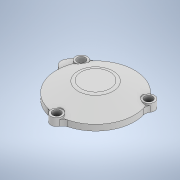
# Autodesk Inventor part: 64. Крышка подшипника
Saved by Autodesk Inventor 2021 (Build 250183000, 183)
## iProperties
Created: 2021-03-10
Part Number: 64. Крышка подшипника
Material: Типовые
Document SubType Name: Modeling
Designer: Данил
Density: 1 g/cm^3
Appearance: По умолчанию
Author: Данил
Autodesk Inventor part; units mm, degrees
ref_plane "YZ Plane" through (0, 0, 0) normal (1, 0, 0) x (0, 1, 0)
ref_plane "XZ Plane" through (0, 0, 0) normal (0, 1, 0) x (-1, 0, 0)
ref_plane "XY Plane" through (0, 0, 0) normal (0, 0, 1) x (1, 0, 0)
sketch "Эскиз1" plane through (0, 0, 0) normal (0, 0, 1) x (1, 0, 0)
  line L0 (0, 11.25) -> (0, -11.25)
  line L1 (-44, -11.25) -> (-44, -8.6)
  line L2 (-42, -6.6) -> (-33.5, -6.6)
  line L3 (-33.5, -6.6) -> (-33.5, -3.25)
  line L4 (-44, -11.25) -> (-53, -11.25)
  line L5 (-53, -11.25) -> (-53, -3.25)
  line L6 (-53, -3.25) -> (-23.9139, 10.3131)
  arc A0 (-42, -6.6) -> (-44, -8.6) centre (-42, -8.6) ccw
  line L7 (-19.6877, 6.75) -> (0, 6.75)
  line L8 (-19.6877, 11.25) -> (0, 11.25)
  arc A1 (-19.6877, 11.25) -> (-23.9139, 10.3131) centre (-19.6877, 1.25) ccw
  line L9 (-30.5721, 1.9039) -> (-24.8078, 5.3398)
  arc A2 (-30.5721, 1.9039) -> (-33.5, -3.25) centre (-27.5, -3.25) ccw
  arc A3 (-19.6877, 6.75) -> (-24.8078, 5.3398) centre (-19.6877, -3.25) ccw
  point P0 (0, 0)
  point P1 (0, 0)
  dimension "d0" = 22.5
  dimension "d1" = 88
  dimension "d2" = 67
  dimension "d3" = 4.65
  dimension "d4" = 2
  dimension "d6" = 8
  dimension "d7" = 106
  dimension "d8" = 25
  dimension "d9" = 4.5
  dimension "d10" = 10
  dimension "d11" = 6
  dimension "d12" = 10
  constraints: 20 end point, 8 point on circle, 8 tangent, 4 centre point, 3 coincident, 3 horizontal, 3 perpendicular, 2 horizontal alignment, 2 vertical, 2 vertical alignment, 1 midpoint
  measures "d0" distance of L0.start L0.end
  measures "d1" diameter of L1 L0
  measures "d2" diameter of L3 L0
  measures "d3" distance between parallel lines of L2 L4
  measures "d4" radius of A0
  measures "d6" distance from line of L4 L5.end
  measures "d7" diameter of L5 L0
  measures "d8" angle of L6 L8
  measures "d9" distance between parallel lines of L7 L8
  measures "d10" radius of A1
  measures "d11" radius of A2
  measures "d12" radius of A3
revolve "Вращение1" add sketch "Эскиз1" angle 360 about axis through (0, 11.25, 0) along (0, -1, 0)
sketch "Эскиз2" plane through (0, -11.25, 0) normal (0, -1, 0) x (1, 0, 0)
  circle A0 centre (0, 0) radius 53 projected
  arc A1 (-13.6119, 51.2222) -> (-7.1912, 56.5052) centre (-16.1802, 60.8868) ccw
  arc A2 (7.1912, 56.5052) -> (13.6119, 51.2222) centre (16.1802, 60.8868) ccw
  circle A3 centre (0, 53) radius 8
  arc A4 (51.1657, -13.8229) -> (52.5306, -22.0249) centre (60.8196, -16.4309) ccw
  arc A5 (45.3394, -34.4804) -> (37.5538, -37.3994) centre (44.6394, -44.4559) ccw
  circle A6 centre (45.8993, -26.5) radius 8
  line L0 (0, 0) -> (45.8993, -26.5) construction
  line L1 (0, 0) -> (0, 53) construction
  line L2 (0, 0) -> (-45.8993, -26.5) construction
  arc A7 (-37.5538, -37.3994) -> (-45.3394, -34.4804) centre (-44.6394, -44.4559) ccw
  circle A8 centre (-45.8993, -26.5) radius 8
  line L3 (-52.7372, -30.6525) -> (-59.6376, -19.2897)
  arc A9 (-55.6932, -5.2214) -> (-52.9952, -0.7151) centre (-57.9947, -0.7826) ccw
  arc A10 (-55.6932, -5.2214) -> (-59.6376, -19.2897) centre (-51.0903, -14.099) ccw
  point P0 (0, 0)
  point P1 (-49.3651, -19.2897)
  dimension "d14" = 10
  dimension "d15" = 10
  dimension "d16" = 16
  dimension "d17" = 16
  dimension "d18" = 10
  dimension "d19" = 10
  dimension "d20" = 120
  dimension "d21" = 120
  dimension "d22" = 16
  dimension "d24" = 10
  dimension "d25" = 5
  dimension "d26" = 10
  constraints: 21 point on circle, 10 centre point, 8 end point, 8 tangent, 2 coincident, 1 horizontal alignment, 1 vertical, 1 vertical alignment, 18 other
  measures "d14" radius of A2
  measures "d15" radius of A1
  measures "d16" diameter of A3
  measures "d17" diameter of A6
  measures "d18" radius of A4
  measures "d19" radius of A5
  measures "d20" angle of L1 L0
  measures "d21" angle of L2 L1
  measures "d22" diameter of A8
  measures "d24" radius of A7
  measures "d25" radius of A9
  measures "d26" radius of A10
extrude "Выдавливание1" add sketch "Эскиз2" against normal blind 8 contours A0 A3 A2 | A4 A6 A0 | A0 A3 | A6 A0 | A0 A1 A3 | A6 A5 A0 | A0 A8 L3 A10 A9 | A7 A8 A0 | A0 A8 picked at (-0.3302, 55.6013) picked at (48.2395, -27.6825) picked at (-48.1398, -27.8618)
sketch "Эскиз3" plane through (0, -3.25, 0) normal (0, 1, 0) x (1, 0, 0)
  circle A0 centre (0, -53) radius 8
  arc A1 (-7.1912, -56.5052) -> (7.1912, -56.5052) centre (0, -53) ccw projected
  circle A2 centre (45.8993, 26.5) radius 8
  circle A3 centre (-45.8993, 26.5) radius 8
  arc A4 (52.5306, 22.0249) -> (45.3394, 34.4804) centre (45.8993, 26.5) ccw projected
  arc A5 (-45.3394, 34.4804) -> (-52.7372, 30.6525) centre (-45.8993, 26.5) ccw projected
  point P0 (0, 0)
  dimension "d29" = 16
  constraints: 3 centre point, 3 concentric, 2 equal radius
  measures "d29" diameter of A0
extrude "Выдавливание2" add sketch "Эскиз3" along normal blind 2.5
sketch "Эскиз4" plane through (0, -0.75, 0) normal (0, 1, 0) x (1, 0, 0)
  arc A0 (-38.1585, 28.5198) -> (-43.7781, 18.7864) centre (-45.8993, 26.5) ccw projected
  arc A1 (43.7781, 18.7864) -> (38.1585, 28.5198) centre (45.8993, 26.5) ccw projected
  arc A2 (-5.6196, -47.3061) -> (5.6196, -47.3061) centre (0, -53) ccw projected
  arc A3 (-52.7372, 30.6525) -> (-49.3651, 19.2897) centre (-45.8993, 26.5) ccw projected
  circle A4 centre (-45.8993, 26.5) radius 5.5
  circle A5 centre (45.8993, 26.5) radius 5.5
  circle A6 centre (0, -53) radius 5.5
  point P0 (0, 0)
  dimension "d33" = 11
  constraints: 3 centre point, 3 coincident, 2 equal radius
  measures "d33" diameter of A4
extrude "Выдавливание3" cut sketch "Эскиз4" along normal through all both and the other way through all
sketch "Эскиз9" plane through (0, -0.75, 0) normal (0, 1, 0) x (1, 0, 0)
  arc A0 (-1.1637, -47.6245) -> (1.1637, -47.6245) centre (0, -53) ccw projected
  circle A1 centre (0, -53) radius 8
  circle A2 centre (-45.8993, 26.5) radius 5.5 projected
  circle A3 centre (-45.8993, 26.5) radius 8
  circle A4 centre (45.8993, 26.5) radius 5.5 projected
  circle A5 centre (45.8993, 26.5) radius 8
  point P0 (0, 0)
  dimension "d58" = 16
  dimension "d59" = 16
  dimension "d60" = 16
  constraints: 3 centre point, 3 coincident
  measures "d58" diameter of A1
  measures "d59" diameter of A3
  measures "d60" diameter of A5
extrude "Выдавливание9" cut sketch "Эскиз9" along normal blind 10
